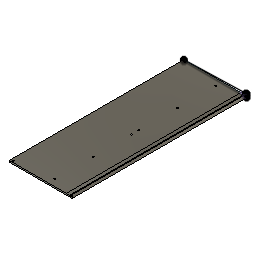
case-bottom (Autodesk Fusion 360 design; units mm, degrees)
part number: 2025-12-03-23-12-50-270
Autodesk Fusion 360 part; units mm, degrees
note: some values were not read from the file. Set by a fixed rule: which sketch regions a step uses.
sketch "Sketch1" plane through (0, 0, 0) normal (0, 1, 0) x (1, 0, 0)
  line L0 (0, 0) -> (-127.2538, 0)
  line L1 (-127.2538, 0) -> (-127.2538, -15.6248)
  line L2 (-127.2538, -15.6248) -> (0, 0)
  line L3 (-127.2538, 0) -> (-0.0202, 0)
  line L4 (0, 0) -> (-0.8531, 6.9478)
  line L5 (-0.8531, 6.9478) -> (-127.2538, -8.5722)
  line L6 (-127.2538, 6.9478) -> (-127.2538, -15.6248)
  line L7 (-127.2538, -8.5722) -> (-126.4008, -15.5201)
  line L8 (-0.8531, 6.9478) -> (-127.2538, 6.9478)
  line L9 (-0.8531, 6.9478) -> (0, 6.9478)
  line L10 (0, 6.9478) -> (0, 0)
  line L11 (-127.2538, 3.7478) -> (0, 3.7478)
  line L12 (-127.2538, 0.7478) -> (-56.2538, 0.7478)
  line L13 (-127.2538, 6.9478) -> (-128.8538, 6.9478)
  line L14 (0, 6.9478) -> (1.6, 6.9478)
  line L15 (1.6, 6.9478) -> (1.6, 0.1989)
  line L16 (-0.0202, 0) -> (1.6, 0.1989)
  line L17 (-128.8538, 6.9478) -> (-128.8538, -15.8213)
  line L18 (-127.2538, -15.6248) -> (-128.8538, -15.8213)
  line L19 (-0.6093, 4.9627) -> (-127.0101, -10.5573)
  line L20 (-87.2538, -3.6609) -> (-87.2538, 3.7478)
  line L21 (-56.2538, 3.7478) -> (-56.2538, 0.7478)
  line L22 (-127.2538, 3.7478) -> (-128.8538, 3.7478)
  circle A0 centre (-41.0275, 0) radius 2.1736
  dimension "d2" = 7
  dimension "d7" = 7
  dimension "d16" = 127.35
  dimension "d17" = 3.2
  dimension "d18" = 71
  dimension "d19" = 1.6
  dimension "d20" = 1.6
  dimension "d21" = 2
  dimension "d28" = 40
  dimension "d29" = 3
  constraint coincident L0.start L2.end
  constraint horizontal L0
  constraint perpendicular L0 L1
  constraint horizontal L3
  constraint perpendicular L2 L4
  constraint coincident L1 L5.end
  constraint perpendicular L4 L5
  constraint coincident L2 L7.end
  constraint perpendicular L2 L7
  constraint coincident L6 L8.end
  constraint perpendicular L6 L8
  constraint vertical L6
  constraint parallel L8 L9
  constraint perpendicular L0 L10
  constraint coincident L6 L11.start
  constraint coincident L10 L11.end
  constraint perpendicular L10 L11
  constraint coincident L6 L12.start
  constraint perpendicular L6 L12
  constraint perpendicular L6 L13
  constraint perpendicular L10 L14
  constraint perpendicular L14 L15
  constraint coincident L15 L16.end
  constraint parallel L2 L16
  constraint perpendicular L13 L17
  constraint coincident L17 L18.end
  constraint parallel L2 L18
  constraint coincident L4 L19.start
  constraint coincident L7 L19.end
  constraint perpendicular L7 L19
  constraint coincident L5 L20.start
  constraint coincident L11 L20.end
  constraint perpendicular L11 L20
  constraint coincident L11 L21.start
  constraint perpendicular L12 L21
  constraint coincident L17 L22.end
  constraint perpendicular L17 L22
  constraint coincident L0 A0.centre
  constraint coincident L19 A0.centre
  measures "d2" angle of L0 L2
  measures "d7" distance of L0.start L4.end
  measures "d16" distance of L4 L7
  measures "d17" distance of L8 L11
  measures "d18" distance of L12.start L12.end
  measures "d19" distance of L6.start L13.end
  measures "d20" distance of L9.end L14.end
  measures "d21" distance of L5 L19
  measures "d28" distance of L1 L20
  measures "d29" distance of L11 L12
extrude "Extrude1" add sketch "Sketch1" along normal blind 362.2 contours L4 L10 L11 | L10 L14 L15 L16 | L4 L9 L10 L11 | L4 L5 L11 L19 | L5 L6 L8 L11 | L6 L13 L17 L22
sketch "Sketch2" plane through (0, 362.2, 0) normal (0, 1, 0) x (-1, 0, 0)
  line L0 (128.8538, -3.7478) -> (10.504, -3.7478)
  line L1 (0.0003, -0.0024) -> (-1.6, -0.1989)
  line L2 (-1.6, -0.1989) -> (-1.6, -6.9478)
  line L3 (-1.6, -6.9478) -> (128.8538, -6.9478)
  line L4 (128.8538, -6.9478) -> (128.8538, -3.7478)
  line L5 (0.0003, -0.0024) -> (-1.6, -0.1989)
  line L6 (-1.6, -0.1989) -> (-1.6, -6.9478)
  line L7 (-1.6, -6.9478) -> (128.8538, -6.9478)
  line L8 (128.8538, -6.9478) -> (128.8538, -3.7478)
  line L9 (128.8538, -3.7478) -> (0.0003, -0.0024)
  line L10 (0.6093, -4.9627) -> (0.0003, -0.0024)
  line L11 (10.504, -3.7478) -> (0.6093, -4.9627)
  constraint coincident L1.start L5.start
  constraint coincident L1.end L2.start
  constraint coincident L2.end L3.start
  constraint coincident L3.end L4.start
  constraint coincident L0.start L4.end
sketch "Sketch3" plane through (0, 0, -6.9478) normal (0, 0, -1) x (1, 0, 0)
  line L0 (1.6, 0) -> (-128.8538, 0)
  line L1 (-128.8538, 0) -> (-128.8538, -362.2)
  line L2 (-128.8538, -362.2) -> (1.6, -362.2)
  line L3 (1.6, -362.2) -> (1.6, 0)
  line L4 (1.6, -362.2) -> (-128.8538, -362.2)
  line L5 (-128.8538, -362.2) -> (-128.8538, 0)
  line L6 (-128.8538, 0) -> (1.6, 0)
  line L7 (1.6, 0) -> (1.6, -362.2)
  circle A0 centre (-124.0538, -3.2) radius 1.55
  circle A1 centre (-3.2, -3.2) radius 1.55
  circle A2 centre (-3.2, -359) radius 1.55
  circle A3 centre (-124.0538, -359) radius 1.55
  line L8 (-48.641, 0) -> (-48.641, -362.2)
  line L9 (-128.8538, -181.1) -> (1.6, -181.1)
  line L10 (-48.641, -268.45) -> (1.6, -268.45)
  circle A4 centre (-48.641, -268.45) radius 1.55
  circle A5 centre (-48.641, -348.187) radius 1.55
  line L11 (-128.8538, -362.2) -> (-0.0003, -362.2)
  circle A6 centre (-48.641, -188.713) radius 1.55
  circle A7 centre (-48.641, -173.487) radius 1.55
  line L12 (-48.641, -93.75) -> (1.6, -93.75)
  circle A8 centre (-48.641, -93.75) radius 1.55
  circle A9 centre (-48.641, -14.013) radius 1.55
  line L13 (-127.2538, 0) -> (0, 0)
  dimension "d30" = 3.1
  dimension "d31" = 3.2
  dimension "d32" = 4.8
  dimension "d33" = 3.1
  dimension "d34" = 4.8
  dimension "d35" = 3.2
  dimension "d36" = 3.1
  dimension "d37" = 4.8
  dimension "d38" = 3.2
  dimension "d39" = 3.1
  dimension "d40" = 4.8
  dimension "d41" = 3.2
  dimension "d43" = 181.1
  dimension "d44" = 87.35
  dimension "d45" = 50.241
  dimension "d46" = 3.1
  dimension "d47" = 3.1
  dimension "d48" = 14.013
  dimension "d49" = 3.1
  dimension "d50" = 7.613
  dimension "d51" = 3.1
  dimension "d52" = 7.613
  dimension "d53" = 87.35
  dimension "d54" = 3.1
  dimension "d55" = 3.1
  dimension "d56" = 14.013
  constraint horizontal L4
  constraint vertical L5
  constraint horizontal L6
  constraint vertical L7
  constraint coincident L0.end L1.start
  constraint coincident L2.end L3.start
  constraint coincident L0 L8.start
  constraint coincident L4 L8.end
  constraint perpendicular L4 L8
  constraint coincident L5 L9.start
  constraint coincident L7 L9.end
  constraint perpendicular L7 L9
  constraint coincident L8 L10.start
  constraint coincident L7 L10.end
  constraint perpendicular L7 L10
  constraint coincident L10.start A4.centre
  constraint coincident L8 A5.centre
  constraint coincident L8 A6.centre
  constraint coincident L8 A7.centre
  constraint coincident L8 L12.start
  constraint coincident L7 L12.end
  constraint perpendicular L7 L12
  constraint coincident L12.start A8.centre
  constraint coincident L8 A9.centre
  measures "d30" diameter of A0
  measures "d31" distance of L6 A0.centre
  measures "d32" distance of L5 A0.centre
  measures "d33" diameter of A1
  measures "d34" distance of L7 A1.centre
  measures "d35" distance of L6 A1.centre
  measures "d36" diameter of A2
  measures "d37" distance of L7 A2.centre
  measures "d38" distance of L4 A2.centre
  measures "d39" diameter of A3
  measures "d40" distance of L5 A3.centre
  measures "d41" distance of L4 A3.centre
  measures "d43" distance of L4 L9
  measures "d44" distance of L9 L10
  measures "d45" distance of L7 L8
  measures "d46" diameter of A4
  measures "d47" diameter of A5
  measures "d48" distance of A5.centre L11
  measures "d49" diameter of A6
  measures "d50" distance of L9 A6.centre
  measures "d51" diameter of A7
  measures "d52" distance of L9 A7.centre
  measures "d53" distance of L9 L12
  measures "d54" diameter of A8
  measures "d55" diameter of A9
  measures "d56" distance of A9.centre L13
hole "Hole1" at (-48.641, 173.487, -6.9478) direction (0, 0, 1) diameter 3.1 end through all
hole "Hole2" at (-48.641, 348.187, -6.9478) direction (0, 0, 1) diameter 3.1 end through all
hole "Hole3" at (-48.641, 268.45, -6.9478) direction (0, 0, 1) diameter 3.1 end through all
hole "Hole4" at (-48.641, 188.713, -6.9478) direction (0, 0, 1) diameter 3.1 end through all
hole "Hole5" at (-48.641, 93.75, -6.9478) direction (0, 0, 1) diameter 3.1 end through all
hole "Hole6" at (-48.641, 14.013, -6.9478) direction (0, 0, 1) diameter 3.1 end through all
hole "Hole7" at (-3.2, 359, -6.9478) direction (0, 0, 1) diameter 3.1 end through all
hole "Hole8" at (-124.0538, 359, -6.9478) direction (0, 0, 1) diameter 3.1 end through all
hole "Hole9" at (-3.2, 3.2, -6.9478) direction (0, 0, 1) diameter 3.1 end through all
hole "Hole10" at (-124.0538, 3.2, -6.9478) direction (0, 0, 1) diameter 3.1 end through all
